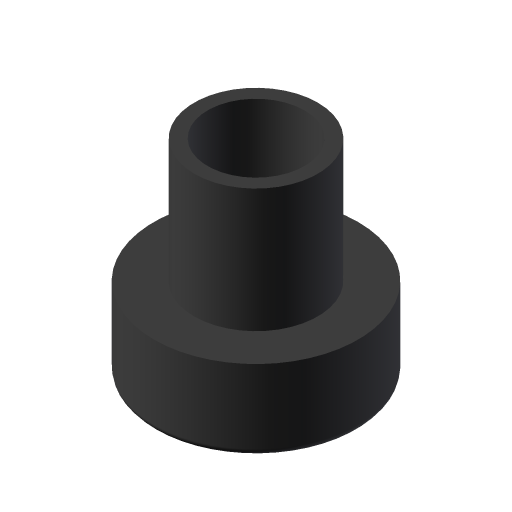
# Autodesk Inventor part: scoringelement
Saved by Autodesk Inventor 2023 (Build 270158000, 158)
## iProperties
Created: 2022-11-04
Part Number: scoringelement
Material: Generic
Document SubType Name: Modeling
Designer: myan
Density: 1 g/cm^3
Appearance: Default
Author: myan
Autodesk Inventor part; units mm, degrees
ref_plane "YZ Plane" through (0, 0, 0) normal (1, 0, 0) x (0, 1, 0)
ref_plane "XZ Plane" through (0, 0, 0) normal (0, 1, 0) x (-1, 0, 0)
ref_plane "XY Plane" through (0, 0, 0) normal (0, 0, 1) x (1, 0, 0)
sketch "Sketch3" plane through (0, 0, 0) normal (1, 0, 0) x (0, 1, 0)
  line L0 (104.7527, -49.0706) -> (47.1264, -49.0706)
  line L1 (46.3327, -49.0706) -> (46.3327, -55.4206)
  line L2 (46.3327, -55.4206) -> (104.7527, -55.4206)
  line L3 (104.7527, -55.4206) -> (104.7527, -49.0706)
  line L4 (117.2485, -26.2106) -> (31.2073, -26.2106)
  line L5 (46.3327, -49.0706) -> (46.3327, -74.4706)
  line L6 (46.3327, -74.4706) -> (11.4077, -74.4706)
  line L7 (9.9136, -68.4942) -> (45.6323, -49.4442)
  arc A0 (9.9136, -68.4942) -> (11.4077, -74.4706) centre (11.4077, -71.2956) ccw
  arc A1 (47.1264, -49.0706) -> (45.6323, -49.4442) centre (47.1264, -52.2456) ccw
  point P0 (0, 0)
  point P1 (46.3327, -55.4206)
  point P2 (64.2516, -56.2504)
  point P3 (46.3327, -49.1714)
  dimension "d13" = 58.42
  dimension "d14" = 6.35
  dimension "d15" = 19.05
  dimension "d17" = 48.26
  dimension "d35" = 3.175
  dimension "d36" = 38.1
  dimension "d37" = 3.175
  constraints: 16 end point, 4 point on circle, 4 tangent, 2 centre point, 2 horizontal, 2 parallel, 2 perpendicular, 2 point on line, 1 vertical
  measures "d13" distance of L1.end L2.end
  measures "d14" distance of L1.start L1.end
  measures "d15" distance between parallel lines of L2 L6
  measures "d17" distance between parallel lines of L4 L6
  measures "d35" radius of A0
  measures "d37" radius of A1
revolve "Revolution2" add sketch "Sketch3" angle 360 about axis through (0, 117.2485, -26.2106) along (0, -1, 0)
body "Solid2"
